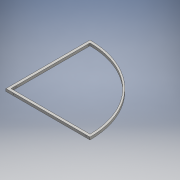
# Autodesk Inventor part: Corner glass holding bar
Saved by Autodesk Inventor 2016 (Build 200138000, 138)
## iProperties
Created: 2015-11-20
Part Number: Corner glass holding bar
Material: 常规
Document SubType Name: Modeling
Designer: Shawn Shi Feng
Density: 1 g/cm^3
Appearance: 默认
Author: Shawn Shi Feng
Autodesk Inventor part; units mm, degrees
ref_plane "YZ Plane" through (0, 0, 0) normal (1, 0, 0) x (0, 1, 0)
ref_plane "XZ Plane" through (0, 0, 0) normal (0, 1, 0) x (-1, 0, 0)
ref_plane "XY Plane" through (0, 0, 0) normal (0, 0, 1) x (1, 0, 0)
sketch "草图1" plane through (0, 0, 0) normal (0, 0, 1) x (1, 0, 0)
  line L0 (-265.6529, 246.0806) -> (-265.6529, -253.9194)
  line L1 (-265.6529, -253.9194) -> (234.3471, -253.9194)
  line L2 (-250.6529, -238.9194) -> (-250.6529, 231.0806)
  line L3 (-250.6529, -238.9194) -> (219.3471, -238.9194)
  arc A0 (219.3471, -238.9194) -> (-250.6529, 231.0806) centre (-250.6529, -238.9194) ccw
  arc A1 (234.3471, -253.9194) -> (-265.6529, 246.0806) centre (-265.6529, -253.9194) ccw
  point P0 (0, 0)
  dimension "d0" = 500
  dimension "d1" = 500
  dimension "d2" = 15
  dimension "d3" = 15
  dimension "d4" = 470
  dimension "d5" = 470
  dimension "d6" = 470
  dimension "d7" = 500
  constraints: 8 end point, 4 point on circle, 2 centre point, 2 vertical, 1 parallel, 1 perpendicular
  measures "d0" distance of L0.start L0.end
  measures "d1" distance of L0.end L1.end
  measures "d2" distance between parallel lines of L0 L2
  measures "d3" distance between parallel lines of L1 L3
  measures "d4" distance of L2.start L3.end
  measures "d5" distance of L2.start L2.end
  measures "d6" radius of A0
  measures "d7" radius of A1
extrude "拉伸1" add sketch "草图1" along normal blind 15
sketch "草图2" plane through (-250.6529, -238.9194, 0) normal (1, 0, 0) x (0, 0, -1)
  circle A0 centre (-7.5, 30) radius 2.5
  circle A1 centre (-7.5, 460) radius 2.5
  line L0 (0, 0) -> (-15, 0) projected
  line L1 (0, 470) -> (0, 0) projected
  point P0 (0, 238.9194)
  dimension "d10" = 5
  dimension "d11" = 5
  dimension "d12" = 30
  dimension "d13" = 430
  dimension "d20" = 7.5
  dimension "d21" = 7.5
  constraints: 2 centre point
  measures "d10" diameter of A0
  measures "d11" diameter of A1
  measures "d12" distance from line of A0.centre L0
  measures "d13" distance of A1.centre A0.centre
  measures "d20" distance from line of L1 A1.centre
  measures "d21" distance from line of L1 A0.centre
extrude "拉伸2" cut sketch "草图2" against normal blind 430
thread "螺纹1" size "M5x0.8" class "6H" standard "ANSI Metric M Profile" full length
thread "螺纹2" size "M5x0.8" class "6H" standard "ANSI Metric M Profile" full length
sketch "草图3" plane through (-250.6529, -238.9194, 0) normal (0, 1, 0) x (1, 0, 0)
  circle A0 centre (30, -7.5) radius 2.5
  circle A1 centre (460, -7.5) radius 2.5
  line L0 (0, 0) -> (0, -15) projected
  line L1 (470, -15) -> (0, -15) projected
  point P0 (250.6529, 0)
  dimension "d22" = 5
  dimension "d23" = 5
  dimension "d24" = 30
  dimension "d25" = 430
  dimension "d26" = 7.5
  dimension "d27" = 7.5
  constraints: 2 centre point
  measures "d22" diameter of A1
  measures "d23" diameter of A0
  measures "d24" distance from line of L0 A0.centre
  measures "d25" distance of A0.centre A1.centre
  measures "d26" distance from line of L1 A1.centre
  measures "d27" distance from line of L1 A0.centre
extrude "拉伸3" cut sketch "草图3" against normal through all
thread "螺纹3" size "M5x0.8" class "6H" standard "ANSI Metric M Profile" full length
thread "螺纹4" size "M5x0.8" class "6H" standard "ANSI Metric M Profile" full length
equation "\"d14\" = d13"
equation "\"d28\" = d22"
